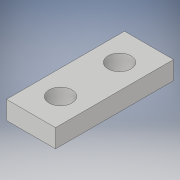
# Autodesk Inventor part: BracketOfTheBracket
Saved by Autodesk Inventor 2019 (Build 230136000, 136)
## iProperties
Created: 2019-06-19
Part Number: BracketOfTheBracket
Material: Generic
Document SubType Name: Modeling
Designer: abdel
Density: 1 g/cm^3
Appearance: Default
Author: abdel
Autodesk Inventor part; units mm, degrees
ref_plane "YZ Plane" through (0, 0, 0) normal (1, 0, 0) x (0, 1, 0)
ref_plane "XZ Plane" through (0, 0, 0) normal (0, 1, 0) x (-1, 0, 0)
ref_plane "XY Plane" through (0, 0, 0) normal (0, 0, 1) x (1, 0, 0)
sketch "Sketch1" plane through (0, 0, 0) normal (0, 1, 0) x (-1, 0, 0)
  line L0 (19.05, 22.8956) -> (38.1, 22.8956)
  line L1 (38.1, 22.8956) -> (19.05, 22.8956)
  line L2 (19.05, -22.8956) -> (38.1, -22.8956)
  line L3 (38.1, -22.8956) -> (38.1, 22.8956)
  line L4 (38.1, 22.8956) -> (19.05, 22.8956)
  line L5 (19.05, 22.8956) -> (19.05, -22.8956)
  line L6 (38.1, 22.8956) -> (28.575, 22.8956)
  circle A0 centre (28.575, 11.4465) radius 4.445
  circle A1 centre (28.575, -11.4516) radius 4.445
  dimension "d6" = 45.7911
  dimension "d7" = 19.05
  dimension "d8" = 19.05
  dimension "d9" = 9.525
  dimension "d13" = 8.89
  constraints: 14 end point, 2 centre point, 2 horizontal, 1 midpoint, 1 parallel, 1 perpendicular
  measures "d6" distance of L2.end L0.end
  measures "d7" distance of L2.start L2.end
  measures "d8" distance of L0.start L0.end
  measures "d9" distance of L0.end L6.end
  measures "d13" diameter of A0
extrude "Extrusion1" add sketch "Sketch1" along normal blind 7.112
body "Solid1"
